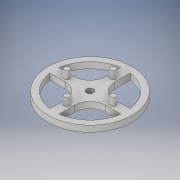
# Autodesk Inventor part: planetaryGearMt
Saved by Autodesk Inventor 2019 (Build 230136000, 136)
## iProperties
Created: 2019-10-26
Part Number: planetaryGearMt
Material: Generic
Document SubType Name: Modeling
Designer: test
Density: 1 g/cm^3
Appearance: Default
Author: test
Autodesk Inventor part; units mm, degrees
ref_plane "YZ Plane" through (0, 0, 0) normal (1, 0, 0) x (0, 1, 0)
ref_plane "XZ Plane" through (0, 0, 0) normal (0, 1, 0) x (-1, 0, 0)
ref_plane "XY Plane" through (0, 0, 0) normal (0, 0, 1) x (1, 0, 0)
sketch "Sketch1" plane through (0, 0, 0) normal (0, 1, 0) x (-1, 0, 0)
  circle A0 centre (0, 19.05) radius 2.2225
  circle A1 centre (-19.05, 0) radius 2.2225
  circle A2 centre (0, -19.05) radius 2.2225
  circle A3 centre (19.05, 0) radius 2.2225
  line L0 (0.635, 24.639) -> (-0.635, 24.639)
  line L1 (-0.635, -24.0273) -> (0.635, -24.0273)
  line L2 (0, 0) -> (0, 2.5439)
  line L3 (28.1077, 0) -> (28.1077, -0.635)
  line L4 (-24.0273, -0.635) -> (-24.0273, 0.635)
  line L5 (3.81, -20.8523) -> (3.81, -16.51)
  line L6 (3.81, 16.51) -> (3.81, 21.464)
  line L7 (-20.8523, 3.81) -> (-16.51, 3.81)
  line L8 (16.51, 3.81) -> (24.9327, 3.81)
  line L9 (-3.81, 21.464) -> (-3.81, 16.51)
  line L10 (-3.81, -16.51) -> (-3.81, -20.8523)
  line L11 (24.9327, -3.81) -> (16.51, -3.81)
  line L12 (-16.51, -3.81) -> (-20.8523, -3.81)
  arc A4 (3.81, 16.51) -> (16.51, 3.81) centre (16.51, 16.51) ccw
  arc A5 (16.51, -3.81) -> (3.81, -16.51) centre (16.51, -16.51) ccw
  arc A6 (-16.51, 3.81) -> (-3.81, 16.51) centre (-16.51, 16.51) ccw
  arc A7 (-3.81, -16.51) -> (-16.51, -3.81) centre (-16.51, -16.51) ccw
  line L13 (0, -3.81) -> (0, 0)
  line L14 (0, 0) -> (0, 3.81)
  line L15 (0, 3.81) -> (0, 0)
  line L16 (3.81, -29.464) -> (3.81, -16.51)
  line L17 (16.51, 3.81) -> (29.464, 3.81)
  line L18 (21.2725, 0) -> (16.8275, 0)
  line L19 (29.464, 3.81) -> (16.51, 3.81)
  line L20 (29.464, -3.81) -> (16.51, -3.81)
  line L21 (0, -3.81) -> (3.81, -3.81)
  line L22 (16.51, -3.81) -> (29.464, -3.81)
  line L23 (3.81, 29.464) -> (3.81, 16.51)
  line L24 (-3.81, 29.464) -> (-3.81, 16.51)
  line L25 (-29.464, 3.81) -> (-16.51, 3.81)
  line L26 (-29.464, -3.81) -> (-16.51, -3.81)
  line L27 (-3.81, -16.51) -> (-3.81, -29.464)
  circle A8 centre (0, 0) radius 34.544
  arc A9 (29.2166, 3.81) -> (3.81, 29.2166) centre (0, 0) ccw
  arc A10 (-3.81, 29.2166) -> (-29.2166, 3.81) centre (0, 0) ccw
  arc A11 (-29.2166, -3.81) -> (-3.81, -29.2166) centre (0, 0) ccw
  arc A12 (3.81, -29.2166) -> (29.2166, -3.81) centre (0, 0) ccw
  point P0 (19.05, 0)
  point P1 (0, -19.05)
  point P2 (29.464, 0)
  point P3 (0, -29.464)
  dimension "d3" = 360
  dimension "d5" = 4.445
  dimension "d8" = 360
  constraints: 56 end point, 18 point on circle, 13 centre point, 10 point on line, 8 parallel, 8 tangent, 4 perpendicular, 3 coincident, 3 equal radius, 3 horizontal, 1 vertical, 14 other
  measures "d5" diameter of A0
extrude "Extrusion3" add sketch "Sketch1" along normal blind 5.08
extrude "Extrusion4" add sketch "Sketch1" along normal blind 11.43 contours A0 | A1 | A2 | L18 A3 | A3 L18
sketch "Sketch2" plane through (0, 5.08, 0) normal (0, 1, 0) x (1, 0, 0)
  circle A0 centre (0, 0) radius 2.8575
  dimension "d26" = 5.715
  constraints: 1 centre point, 1 coincident
  measures "d26" diameter of A0
extrude "Extrusion5" cut sketch "Sketch2" against normal blind 11.43
body "Solid2"
